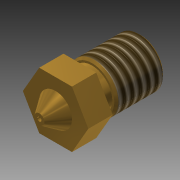
# Autodesk Inventor part: nozzle-0,6
Saved by Autodesk Inventor 2015 (Build 190159000, 159)
## iProperties
Created: 2015-02-05
Part Number: nozzle-0,6
Material: Типовые
Document SubType Name: Modeling
Designer: Parabolik
Density: 1 g/cm^3
Appearance: Латунь - сатинированная
Author: Parabolik
Autodesk Inventor part; units mm, degrees
ref_plane "YZ Plane" through (0, 0, 0) normal (1, 0, 0) x (0, 1, 0)
ref_plane "XZ Plane" through (0, 0, 0) normal (0, 1, 0) x (-1, 0, 0)
ref_plane "XY Plane" through (0, 0, 0) normal (0, 0, 1) x (1, 0, 0)
sketch "Эскиз1" plane through (0, 0, 0) normal (0, 0, 1) x (1, 0, 0)
  line L0 (0, 0) -> (0, 15)
  line L1 (0, 12.5) -> (3, 12.5)
  line L2 (2.0254, 2) -> (4.0415, 2)
  line L3 (2.5, 5) -> (4.0415, 5)
  line L4 (2.5, 6.5) -> (3, 6.5)
  line L5 (0, 0) -> (0.625, 0)
  line L6 (2.5, 6.5) -> (2.5, 5)
  line L7 (3, 12.5) -> (3, 6.5)
  line L8 (0.625, 0) -> (2.0254, 2)
  line L9 (4.0415, 5) -> (4.0415, 2)
  line L10 (0, 12.5) -> (0, 0)
  dimension "d0" = 15
  dimension "d1" = 12.5
  dimension "d2" = 10.5
  dimension "d3" = 7.5
  dimension "d4" = 6
  dimension "d6" = 5
  dimension "d7" = 6
  dimension "d8" = 125
  dimension "d11" = 8.083
  dimension "d44" = 1.25
  constraints: 22 end point, 4 horizontal, 3 perpendicular, 1 collinear, 1 point on line, 1 vertical
  measures "d0" distance of L0.start L0.end
  measures "d1" distance from line of L0.start L1
  measures "d2" distance between parallel lines of L2 L1
  measures "d3" distance between parallel lines of L3 L1
  measures "d4" distance between parallel lines of L4 L1
  measures "d6" diameter of L6 L0
  measures "d7" diameter of L7 L0
  measures "d8" angle of L8 L2
  measures "d11" diameter of L9 L0
  measures "d44" diameter of L5.end L0
revolve "Вращение1" add sketch "Эскиз1" angle 360 about axis through (0, 0, 0) along (0, 1, 0)
chamfer "Фаска1" distance 0.25 angle 45 2 edges at (-3, 12.5, 0) (-3, 6.5, 0)
thread "Резьба1" size "M6x1" class "6g" standard "ANSI Metric M Profile" full length
sketch "Эскиз2" plane through (0, 12.5, 0) normal (0, 1, 0) x (1, 0, 0)
  point P0 (0, 0)
  point P1 (0, 0)
  constraints: 1 coincident
sketch "Эскиз3" plane through (0, 0, 0) normal (0, -1, 0) x (1, 0, 0)
  point P0 (0, 0)
  point P1 (0, 0)
  constraints: 1 coincident
hole "Отверстие1" at (0, 12.5, 0) direction (0, -1, 0) diameter 1.5 depth 11.5 tip angle 130
hole "Отверстие2" at (0, 12.5, 0) direction (0, -1, 0) diameter 2 depth 10.4 tip angle 130
chamfer "Фаска2" distance 0.2 angle 45 1 edges at (0, 12.5, -1)
hole "Отверстие3" at (0, 0, 0) direction (0, 1, 0) diameter 0.5 depth 1
sketch "Эскиз4" plane through (0, 2, 0) normal (0, -1, 0) x (1, 0, 0)
  circle A0 centre (0, 0) radius 0.25 projected
  circle A1 centre (0, 0) radius 4.0415 projected
  line L0 (4.0415, 0) -> (2.0208, -3.5)
  line L1 (2.0208, -3.5) -> (-2.0207, -3.5)
  line L2 (-2.0207, -3.5) -> (-4.0415, 0)
  line L3 (-4.0415, 0) -> (-2.0208, 3.5)
  line L4 (-2.0208, 3.5) -> (2.0207, 3.5)
  line L5 (2.0207, 3.5) -> (4.0415, 0)
  constraints: 12 end point, 1 coincident, 1 horizontal alignment, 14 other
extrude "Выдавливание1" cut sketch "Эскиз4" against normal blind 3 contours L5 A1 | A1 L0 | L4 A1 | A1 L1 | L3 A1 | A1 L2
